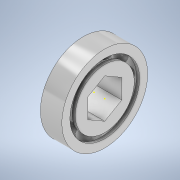
# Autodesk Inventor part: rodamientov2
Saved by Autodesk Inventor 2020.3 (Build 243373000, 373)
## iProperties
Created: 2020-12-04
Part Number: rodamientov2
Material: Generic
Document SubType Name: Modeling
Designer: Yu Jinyu
Density: 1 g/cm^3
Appearance: Aluminum - Dark
Author: Yu Jinyu
Autodesk Inventor part; units mm, degrees
ref_plane "YZ Plane" through (0, 0, 0) normal (1, 0, 0) x (0, 1, 0)
ref_plane "XZ Plane" through (0, 0, 0) normal (0, 1, 0) x (-1, 0, 0)
ref_plane "XY Plane" through (0, 0, 0) normal (0, 0, 1) x (1, 0, 0)
sketch "Sketch1" plane through (0, 0, 0) normal (0, 0, 1) x (1, 0, 0)
  line L0 (-4, 16) -> (4, 16)
  line L1 (4, 16) -> (4, 13)
  line L2 (-4, 13) -> (-4, 16)
  line L3 (-4, 16) -> (4, 13) construction
  line L4 (4, 16) -> (-4, 13) construction
  line L5 (-4, 11) -> (-4, 8)
  line L6 (-4, 8) -> (4, 8)
  line L7 (4, 8) -> (4, 11)
  line L8 (4, 11) -> (-4, 8) construction
  line L9 (-4, 11) -> (4, 8) construction
  line L10 (4, 13) -> (2.8284, 13)
  line L11 (-2.8284, 13) -> (-4, 13)
  line L12 (4, 11) -> (2.8284, 11)
  line L13 (-2.8284, 11) -> (-4, 11)
  arc A0 (2.8284, 13) -> (-2.8284, 13) centre (0, 12) ccw
  arc A1 (-2.8284, 11) -> (2.8284, 11) centre (0, 12) ccw
  line L14 (0, 14.5) -> (0, 15)
  line L15 (0, 0) -> (0, 8)
  line L16 (0, 9) -> (0, 9.5)
  line L17 (-5.6, 0) -> (5.6, 0) projected
  point P0 (0, 14.5)
  point P1 (0, 9.5)
  dimension "d6" = 8
  dimension "d7" = 3
  dimension "d8" = 8
  dimension "d9" = 3
  dimension "d11" = 8
  constraints: 34 end point, 6 parallel, 6 point on circle, 5 midpoint, 3 horizontal, 3 perpendicular, 3 vertical, 2 centre point
  measures "d6" distance of L1.end L2.start
  measures "d7" distance of L0.end L1.end
  measures "d8" distance of L6.end L5.end
  measures "d9" distance of L6.end L7.end
  measures "d11" distance from line of L15.start L6
sketch "Sketch2" plane through (0, 0, 0) normal (1, 0, 0) x (0, 1, 0)
  point P0 (0, 0)
revolve "Revolution1" add sketch "Sketch1" angle 360 about axis through (-10, 0, 0) along (1, 0, 0)
sketch "Sketch5" plane through (0, 0, 0) normal (1, 0, 0) x (0, 1, 0)
  point P0 (0, 0)
sketch "Sketch6" plane through (0, 0, 0) normal (0, 0, 1) x (1, 0, 0)
  point P0 (0, 0)
sketch "Sketch7" plane through (4, 0, 0) normal (1, 0, 0) x (0, 0, -1)
  point P0 (0, 0)
sketch "Sketch8" plane through (0, 0, 0) normal (0, 1, 0) x (-1, 0, 0)
  line L0 (4, 16) -> (4, -16) projected
  line L1 (-4, 16) -> (-4, -16) projected
  arc A0 (2.8284, -11) -> (-2.8284, -11) centre (0, -12) ccw projected
  arc A1 (-2.8284, -13) -> (2.8284, -13) centre (0, -12) ccw projected
  arc A2 (-2.8284, -13) -> (2.8284, -13) centre (0, -12) ccw projected
  arc A3 (-2.8284, -13) -> (2.8284, -13) centre (0, -12) ccw projected
  arc A4 (-2.8284, -13) -> (2.8284, -13) centre (0, -12) ccw projected
  arc A5 (3, -12) -> (-3, -12) centre (0, -12) ccw
  arc A6 (0, -9.7) -> (0, -14.3) centre (0, -12) ccw
  line L2 (0, -14.3) -> (0, -9.7)
  line L3 (0, -22.4) -> (0, 22.4) projected
  point P0 (0, 0)
  dimension "d16" = 4.6
  constraints: 4 point on circle, 2 centre point, 2 coincident, 2 end point
  measures "d16" diameter of A6
revolve "Revolution2" add sketch "Sketch8" angle 360 about axis through (0, 0, -10) along (0, 0, 1)
pattern_circular "Circular Pattern1" count 10 over 360 about axis through (-3.4142, 0, 0) along (1, 0, 0) of "Revolution2"
sketch "Sketch9" plane through (0, 0, 0) normal (0, 1, 0) x (-1, 0, 0)
  point P0 (0, 0)
sketch "Sketch10" plane through (4, 0, 0) normal (1, 0, 0) x (0, 0, -1)
  point P0 (0, 0)
sketch "Sketch11" plane through (-4, 0, 0) normal (-1, 0, 0) x (0, 0, 1)
  circle A0 centre (0, 0) radius 8
  constraints: 1 centre point, 1 coincident
extrude "Extrusion1" add sketch "Sketch11" against normal blind 8
sketch "Sketch12" plane through (-4, 0, 0) normal (-1, 0, 0) x (0, 0, 1)
  circle A0 centre (0, 0) radius 7.875
  circle A1 centre (0, 0) radius 11 projected
  line L0 (6.275, -3.7931) -> (-0.1474, -7.3309)
  line L1 (-0.1474, -7.3309) -> (-6.4224, -3.5378)
  line L2 (-6.4224, -3.5378) -> (-6.275, 3.7931)
  line L3 (-6.275, 3.7931) -> (0.1474, 7.3309)
  line L4 (0.1474, 7.3309) -> (6.4224, 3.5378)
  line L5 (6.4224, 3.5378) -> (6.275, -3.7931)
  dimension "d23" = 15.75
  dimension "d24" = 12.7
  constraints: 12 end point, 2 coincident, 1 centre point, 13 other
  measures "d23" diameter of A0
  measures "d24" distance between parallel lines of L1 L4
extrude "Extrusion2" add sketch "Sketch12" along normal blind 3 contours A0 | L0 L1 L2 L3 L4 L5
sketch "Sketch13" plane through (-7, 0, 0) normal (-1, 0, 0) x (0, 0, 1)
  circle A0 centre (0, 0) radius 7.875 projected
  line L0 (0, 7.3323) -> (6.35, 3.6662)
  line L1 (6.35, 3.6662) -> (6.35, -3.6662)
  line L2 (6.35, -3.6662) -> (0, -7.3323)
  line L3 (0, -7.3323) -> (-6.35, -3.6662)
  line L4 (-6.35, -3.6662) -> (-6.35, 3.6662)
  line L5 (-6.35, 3.6662) -> (0, 7.3323)
  dimension "d27" = 12.7
  constraints: 12 end point, 1 coincident, 13 other
  measures "d27" distance between parallel lines of L3 L0
extrude "Extrusion3" cut sketch "Sketch13" against normal blind 11 contours L0 L1 L2 L3 L4 L5
body "Solid1"
